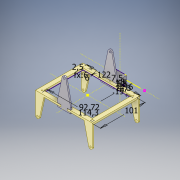
# Autodesk Inventor part: ControllerPCBHolder
Saved by Autodesk Inventor 2019.1 (Build 231200000, 200)
## iProperties
Created: 2018-09-15
Part Number: ControllerPCBHolder
Material: Generisch
Document SubType Name: Modeling
Designer: JochenAlt
Density: 1 g/cm^3
Appearance: Nylon 6
Author: JochenAlt
Autodesk Inventor part; units mm, degrees
ref_plane "YZ Plane" through (0, 0, 0) normal (1, 0, 0) x (0, 1, 0)
ref_plane "XZ Plane" through (0, 0, 0) normal (0, 1, 0) x (-1, 0, 0)
ref_plane "XY Plane" through (0, 0, 0) normal (0, 0, 1) x (1, 0, 0)
sketch "Skizze1" plane through (0, 0, 0) normal (0, 0, 1) x (1, 0, 0)
  line L0 (-61, 50.5) -> (61, 50.5)
  line L1 (61, 50.5) -> (61, -50.5)
  line L2 (61, -50.5) -> (-61, -50.5)
  line L3 (-61, -50.5) -> (-61, 50.5)
  line L4 (0, 70.7) -> (0, -70.7) construction
  line L5 (-85.4, 0) -> (85.4, 0) construction
  line L6 (-55, 44.5) -> (55, 44.5)
  line L7 (55, 44.5) -> (55, -44.5)
  line L8 (55, -44.5) -> (-55, -44.5)
  line L9 (-55, -44.5) -> (-55, 44.5)
  line L10 (-57.15, 46.36) -> (57.15, 46.36) construction
  line L11 (57.15, 46.36) -> (57.15, -46.36) construction
  line L12 (57.15, -46.36) -> (-57.15, -46.36) construction
  line L13 (-57.15, -46.36) -> (-57.15, 46.36) construction
  circle A0 centre (-57.15, 46.36) radius 1.25
  circle A1 centre (57.15, 46.36) radius 1.25
  circle A2 centre (-57.15, -46.36) radius 1.25
  circle A3 centre (57.15, -46.36) radius 1.25
  circle A4 centre (57.15, 46.36) radius 2.8429
  circle A5 centre (-57.15, 46.36) radius 2.8429
  circle A6 centre (-57.15, -46.36) radius 2.8429
  circle A7 centre (57.15, -46.36) radius 2.8429
  point P0 (0, 0)
  dimension "d0" = 122
  dimension "d1" = 101
  dimension "d4" = 6
  dimension "d5" = 6
  dimension "d6" = 2.5
  dimension "d7" = 114.3
  dimension "d8" = 92.72
  constraints: 24 end point, 8 coincident, 6 parallel, 4 centre point, 3 equal radius, 3 horizontal, 3 perpendicular, 18 other
  measures "d0" distance of L0.start L0.end
  measures "d1" distance of L0.end L1.end
  measures "d4" distance between parallel lines of L6 L0
  measures "d5" distance between parallel lines of L9 L3
  measures "d6" diameter of A0
  measures "d7" distance of L11.end L12.end
  measures "d8" distance of L10.end L11.end
extrude "Extrusion2" add sketch "Skizze1" along normal blind 4 contours L0 L1 L2 L3 | A4 | A7 | A6 | A5
extrude "Extrusion15" add sketch "Skizze1" against normal blind 5 contours A4 | A7 | A6 | A5
sketch "Skizze2" plane through (0, 0, 0) normal (0, 1, 0) x (-1, 0, 0)
  arc A0 (55.797, -45.731) -> (64.6888, -44.75) centre (60.1888, -44.75) ccw
  arc A1 (-64.6888, -44.75) -> (-55.797, -45.731) centre (-60.1888, -44.75) ccw
  line L0 (0, -108.2) -> (0, 92.7) construction
  line L1 (-97.3, 0) -> (97.3, 0) construction
  circle A2 centre (60.1888, -44.75) radius 1.75
  circle A3 centre (-60.1888, -44.75) radius 1.75
  line L2 (64.6888, -44.75) -> (64.6888, 4)
  line L3 (-64.6888, -44.75) -> (-64.6888, 4)
  line L4 (-61, 4) -> (61, 4) construction
  line L5 (64.6888, 4) -> (44.6888, 4)
  line L6 (-64.6888, 4) -> (-44.6888, 4)
  circle A4 centre (0, 59.5) radius 1.75
  arc A5 (4.4056, 60.4167) -> (-4.4056, 60.4167) centre (0, 59.5) ccw
  line L7 (60.1888, -44.75) -> (0, 59.5) construction
  line L8 (61, 0) -> (-61, 0) construction
  circle A6 centre (0, -10) radius 69.5 construction
  line L9 (60.1888, -44.75) -> (-60.1888, -44.75) construction
  line L10 (0, 59.5) -> (-60.1888, -44.75) construction
  line L11 (55, 4) -> (-55, 4) construction
  line L12 (7, 0) -> (7, 0)
  line L13 (7, 0) -> (-7, 0)
  line L14 (7, 4.5) -> (15, 4.5)
  line L15 (15, 4.5) -> (15, 9.0368)
  line L16 (-15, 9.0368) -> (-15, 4.5)
  line L17 (-15, 4.5) -> (-7, 4.5)
  line L18 (7, 9.5) -> (-7, 9.5)
  line L19 (7, 9.5) -> (7, 0)
  line L20 (-7, 9.5) -> (-7, 0)
  line L21 (-4.4056, 60.4167) -> (-14.9056, 9.9535)
  line L22 (4.4056, 60.4167) -> (14.9056, 9.9535)
  line L23 (-4.5, 59.3542) -> (-4.5, 59.5)
  arc A7 (-14.9056, 9.9535) -> (-15, 9.0368) centre (-10.5, 9.0368) ccw
  arc A8 (15, 9.0368) -> (14.9056, 9.9535) centre (10.5, 9.0368) ccw
  line L24 (-55.797, -45.731) -> (-44.6888, 4)
  line L25 (55.797, -45.731) -> (44.6888, 4)
  point P0 (0, 0)
  point P1 (15, 9.5)
  dimension "d12" = 3.5
  dimension "d22" = 69.5
  dimension "d23" = 4.5
  dimension "d54" = 5
  dimension "d61" = 30
  dimension "d71" = 0.5
  dimension "d74" = 10
  dimension "d76" = 5
  dimension "d81" = 20
  dimension "d82" = 14
  constraints: 42 end point, 13 point on circle, 11 tangent, 9 centre point, 8 point on line, 6 equal radius, 5 horizontal, 3 coincident, 3 collinear, 3 midpoint, 3 vertical, 2 equal length, 2 perpendicular, 4 other
  measures "d12" diameter of A2
  measures "d22" radius of A6
  measures "d23" radius of A0
  measures "d54" distance of point (15, 9.5) L14.end
  measures "d61" distance between parallel lines of L16 L15
  measures "d71" distance between parallel lines of L11 L14
  measures "d74" distance from line of A6.centre L1
  measures "d76" distance between parallel lines of L18 L17
  measures "d81" distance of L6.end L3.end
  measures "d82" distance of L18.start L18.end
extrude "Extrusion3" add sketch "Skizze2" along normal blind 3 from surface at 50.5 contours L25 L5 L2 A0 | L3 L6 L24 A1
extrude "Extrusion4" add sketch "Skizze2" against normal blind 3 from surface at -50.5 contours L25 L5 L2 A0 | L3 L6 L24 A1
sketch "Skizze4" plane through (0, 0, 0) normal (0, 0, 1) x (1, 0, 0)
  line L0 (-64.6888, 53.5) -> (-64.6888, 50.5) projected
  line L1 (44.6888, -53.5) -> (64.6888, -53.5) projected
  line L2 (-64.6888, 53.5) -> (64.6888, 53.5)
  line L3 (64.6888, 53.5) -> (64.6888, -53.5)
  line L4 (64.6888, -53.5) -> (-64.6888, -53.5)
  line L5 (-64.6888, -53.5) -> (-64.6888, 53.5)
  line L6 (61, -50.5) -> (61, 50.5) projected
  line L7 (61, -50.5) -> (-61, -50.5)
  line L8 (-61, -50.5) -> (-61, 50.5)
  line L9 (-61, 50.5) -> (61, 50.5)
  line L10 (61, 50.5) -> (61, -50.5)
  point P0 (0, 0)
  point P1 (55.6888, -53.5)
  constraints: 16 end point, 4 parallel, 2 horizontal, 2 perpendicular, 1 coincident
extrude "Extrusion5" add sketch "Skizze4" along normal blind 4
extrude "Extrusion7" cut sketch "Skizze2" along normal up to surface (3 mm away) from surface at -53.5 contours A4 | L19 L13 L20 L18
extrude "Extrusion8" cut sketch "Skizze2" against normal up to surface (3 mm away) from surface at 53.5 contours A4 | L19 L13 L20 L18
sketch "Skizze5" plane through (0, 0, 0) normal (0, 1, 0) x (-1, 0, 0)
  point P0 (0, 0)
extrude "Extrusion6" add sketch "Skizze2" against normal up to surface (3 mm away) from surface at -50.5 separate body contours L22 A8 L15 L14 L19 L18 L20 L17 L16 A7 L21 A5 | L19 L13 L20 L18
extrude "Extrusion9" add sketch "Skizze2" against normal up to surface (3 mm away) from surface at 53.5 contours L22 A8 L15 L14 L19 L18 L20 L17 L16 A7 L21 A5 | L19 L13 L20 L18 bodies 2
sketch "Skizze7" plane through (4, -53.5, 0) normal (0, 0, -1) x (-1, 0, 0)
  line L0 (-41.5822, 0) -> (-3, 0) construction
  line L1 (19, 0) -> (19, 0)
  line L2 (-11, 0) -> (-11, 9)
  line L3 (-11, 9) -> (19, 9)
  line L4 (19, 9) -> (19, 0)
  line L5 (59, 9) -> (-51, 9) construction
  line L6 (19, 107) -> (-11, 107)
  line L7 (-11, 107) -> (-11, 98)
  line L8 (-11, 98) -> (19, 98)
  line L9 (19, 98) -> (19, 107)
  line L10 (59, 98) -> (-51, 98) projected
  line L11 (8.4056, 3) -> (8.4056, 0) construction
  line L12 (-0.5, 3) -> (-0.5, 0) construction
  line L13 (2.25, 3) -> (5.75, 3) construction
  line L14 (2.25, 0) -> (5.75, 0) construction
  line L15 (11, 3) -> (-3, 3) construction
  line L16 (4, 3) -> (4, 0) construction
  line L17 (8.4056, 0) -> (-0.4056, 0) construction
  line L18 (19, 9) -> (19, 0)
  line L19 (19, 9) -> (19, 9)
  line L20 (19, 0) -> (-11, 0)
  point P0 (4, 53.5)
  point P1 (11.5, 0)
  point P2 (59.6888, 0)
  point P3 (-3.5, 107)
  point P4 (8.5, 3)
  point P5 (8.5, 0)
  point P6 (11.5, 3)
  point P7 (-51.6888, 0)
  point P8 (11, 3)
  dimension "d45" = 30
  dimension "d51" = 15
  constraints: 24 end point, 7 parallel, 3 horizontal, 3 perpendicular, 2 collinear, 2 point on line, 1 midpoint, 6 other
  measures "d45" distance between parallel lines of L2 L4
  measures "d51" distance between parallel lines of L16 L2
extrude "Extrusion10" add sketch "Skizze7" along normal blind 3 contours L9 L8 L7 L6 bodies 2
extrude "Extrusion12" add sketch "Skizze7" along normal blind 3 contours L2 L3 L4 L20 bodies 2
sketch "Skizze10" plane through (0, 53.5, 59.5) normal (0, 1, 0) x (1, 0, 0)
  line L0 (15, 62.5) -> (-15, 62.5)
  line L1 (-15, 62.5) -> (-15, 50)
  line L2 (-15, 50) -> (15, 50)
  line L3 (15, 50) -> (15, 62.5)
  point P0 (0, 59.5)
  point P1 (-7, 50)
  constraints: 8 end point, 3 perpendicular, 1 coincident, 1 horizontal, 1 point on line
extrude "Extrusion14" add sketch "Skizze10" along normal blind 20 bodies 2
sketch "Skizze6" plane through (-55.6888, 73.5, -5) normal (0, -1, 0) x (1, 0, 0)
  line L0 (-34.8755, 5) -> (146.253, 5) construction
  line L1 (55.6888, 91.65) -> (55.6888, -66.9) construction
  line L2 (44.6888, 2.5) -> (63.6888, 2.5)
  line L3 (63.6888, 2.5) -> (63.6888, -13.5)
  line L4 (63.6888, -13.5) -> (44.6888, -13.5)
  line L5 (44.6888, -13.5) -> (44.6888, 2.5)
  line L6 (101.271, 5) -> (62.6888, 5) projected
  circle A0 centre (47.1888, -11) radius 1.75
  circle A1 centre (61.1888, -11) radius 1.75
  line L7 (61.1888, -11) -> (47.1888, -11) construction
  line L8 (54.1888, 2.5) -> (54.1888, -13.5) construction
  line L9 (42.6888, -15.5) -> (65.6888, -15.5)
  line L10 (65.6888, -15.5) -> (65.6888, 4.5)
  line L11 (65.6888, 4.5) -> (42.6888, 4.5)
  line L12 (42.6888, 4.5) -> (42.6888, -15.5)
  circle A2 centre (61.1888, -11) radius 3.25
  circle A3 centre (47.1888, -11) radius 3.25
  line L13 (42.6888, 4.5) -> (42.6888, 14.5)
  line L14 (42.6888, 14.5) -> (65.6888, 14.5)
  line L15 (65.6888, 14.5) -> (65.6888, 4.5)
  line L16 (40.6888, 14.5) -> (70.6888, 14.5) projected
  point P0 (55.6888, 5)
  point P1 (55.6888, 5)
  point P2 (111.3775, 5)
  point P3 (55.6888, -5)
  dimension "d24" = 19
  dimension "d25" = 16
  dimension "d30" = 3.5
  dimension "d31" = 2.5
  dimension "d32" = 14
  dimension "d33" = 8
  dimension "d48" = 2
  dimension "d58" = 1.5
  dimension "d69" = 7.5
  constraints: 26 end point, 5 perpendicular, 4 centre point, 4 parallel, 2 coincident, 2 equal radius, 2 horizontal, 2 midpoint, 2 point on line, 1 symmetric about line, 1 vertical, 4 other
  measures "d24" distance of L3.end L4.end
  measures "d25" distance of L2.end L3.end
  measures "d30" diameter of A0
  measures "d31" distance from line of L4 L7.start
  measures "d32" distance of L7.start L7.end
  measures "d33" distance between parallel lines of L3 L1
  measures "d48" distance between parallel lines of L4 L9
  measures "d58" radial gap between concentric circles of A2 A1
  measures "d69" distance from line of L2 point (55.689, -5)
extrude "Extrusion11" add sketch "Skizze6" against normal blind 4 contours L2 L3 A2 L4 A3 L5 | A3 L4 L5 | L5 A3 | A2 L3 | L3 A2 L4 | A3 L4 L5 | L3 L4 A2 | L4 A2 | L4 A3 | L12 L11 L10 L9 bodies 2
extrude "Extrusion13" add sketch "Skizze6" against normal blind 4 from surface at -4 contours A3 L4 L5 | L5 A3 | A2 L3 | L3 A2 L4 | L4 A2 | L4 A3 picked at (47.2591, -13.2457) picked at (61.1185, -13.2457) bodies 2
equation "\"d5\" = d4"
